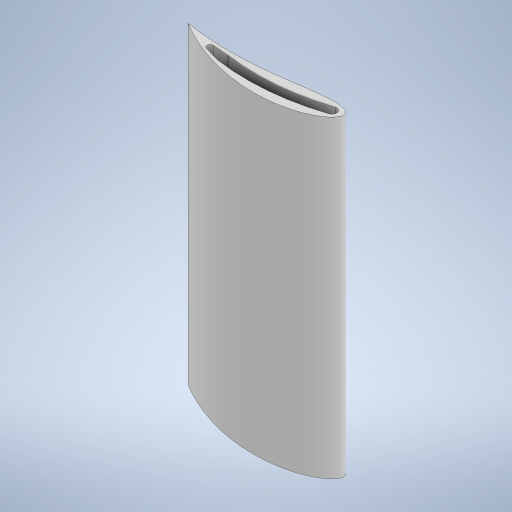
# Autodesk Inventor part: 9518
Saved by Autodesk Inventor 2023 (Build 270158000, 158)
## iProperties
Created: 2023-03-15
Part Number: 9518
Material: 一般
Document SubType Name: Modeling
Designer: USER
Density: 1 g/cm^3
Appearance: 預設
Author: USER
Autodesk Inventor part; units mm, degrees
ref_plane "YZ Plane" through (0, 0, 0) normal (1, 0, 0) x (0, 1, 0)
ref_plane "XZ Plane" through (0, 0, 0) normal (0, 1, 0) x (-1, 0, 0)
ref_plane "XY Plane" through (0, 0, 0) normal (0, 0, 1) x (1, 0, 0)
sketch "草圖1" plane through (0, 0, 0) normal (0, 1, 0) x (-1, 0, 0)
  spline S0 degree 5 poles (50, 0) (50.0018, 0.0049) (49.9549, 0.0322) (49.7247, 0.1379) (49.7279, 0.2103) (49.0894, 0.5065) (48.8341, 0.7267) (48.0356, 1.1334) (47.3779, 1.5287) (46.409, 2.0302) (45.4109, 2.5501) (44.2282, 3.1221) (42.9528, 3.7109) (41.5444, 4.3173) (40.0326, 4.9232) (38.4133, 5.5196) (36.7002, 6.0934) (34.9, 6.6339) (33.0241, 7.1302) (31.0833, 7.572) (29.0901, 7.9505) (27.0573, 8.2573) (24.9994, 8.4858) (22.9309, 8.6309) (20.8674, 8.6883) (18.8247, 8.6569) (16.819, 8.5358) (14.8662, 8.3275) (12.9821, 8.0353) (11.1817, 7.665) (9.4795, 7.2237) (7.8884, 6.7205) (6.42, 6.1652) (5.0847, 5.5689) (3.8908, 4.9431) (2.8449, 4.2994) (1.9517, 3.6485) (1.2135, 3.0004) (0.6319, 2.3616) (0.2072, 1.7375) (-0.0547, 1.1287) (-0.1445, 0.5417) (-0.0431, -0.0146) (0.2327, -0.5065) (0.6667, -0.9034) (1.2361, -1.2172) (1.9287, -1.454) (2.7384, -1.6234) (3.6613, -1.7301) (4.6932, -1.778) (5.8282, -1.7712) (7.0599, -1.7133) (8.3813, -1.6096) (9.7854, -1.4651) (11.2651, -1.2861) (12.8135, -1.0791) (14.4239, -0.8511) (16.0897, -0.6096) (17.8041, -0.3622) (19.5603, -0.1162) (21.3511, 0.121) (23.1691, 0.3426) (25.0059, 0.5429) (26.8531, 0.7166) (28.7012, 0.8597) (30.5403, 0.9698) (32.3598, 1.0451) (34.1488, 1.0857) (35.896, 1.0928) (37.5891, 1.069) (39.2181, 1.0169) (40.7669, 0.9428) (42.2336, 0.8471) (43.5868, 0.7445) (44.856, 0.6222) (45.953, 0.5206) (47.0127, 0.3808) (47.7712, 0.3214) (48.64, 0.1592) (48.9786, 0.1804) (49.6561, 0.0095) (49.7006, 0.0688) (49.9448, 0.0039) (49.9982, -0.0049) (50, 0) knots 0 0 0 0 0 0 0.005631 0.010546 0.017382 0.02568 0.035134 0.045569 0.056859 0.068903 0.081616 0.094923 0.108756 0.123052 0.137755 0.152809 0.168162 0.183765 0.199568 0.215524 0.231585 0.247705 0.263835 0.279929 0.295939 0.311816 0.32751 0.342973 0.358152 0.372996 0.387454 0.401471 0.414995 0.427972 0.440349 0.452078 0.46312 0.473455 0.483105 0.49216 0.500768 0.509124 0.517469 0.526039 0.535015 0.54453 0.554657 0.565407 0.576758 0.588667 0.601088 0.613972 0.627272 0.640942 0.654941 0.669226 0.68376 0.698506 0.713426 0.728485 0.743649 0.75888 0.774142 0.789396 0.804604 0.819723 0.834709 0.849515 0.864091 0.878383 0.892334 0.905881 0.918959 0.931493 0.943401 0.954593 0.96496 0.97437 0.982641 0.989463 0.994372 1 1 1 1 1 1
  point P0 (0, 0)
  point P1 (49.7146, 0.1731)
  point P2 (49.3586, 0.3861)
  point P3 (48.8615, 0.6782)
  point P4 (48.2248, 1.0432)
  point P5 (47.4504, 1.4739)
  point P6 (46.541, 1.9614)
  point P7 (45.4995, 2.496)
  point P8 (44.3301, 3.0669)
  point P9 (43.0373, 3.6629)
  point P10 (41.6267, 4.2721)
  point P11 (40.1046, 4.8827)
  point P12 (38.4784, 5.4828)
  point P13 (36.7563, 6.0603)
  point P14 (34.9477, 6.604)
  point P15 (33.0628, 7.103)
  point P16 (31.1129, 7.5473)
  point P17 (29.1101, 7.9275)
  point P18 (27.0678, 8.2355)
  point P19 (25, 8.4646)
  point P20 (22.9217, 8.6095)
  point P21 (20.8483, 8.6662)
  point P22 (18.7959, 8.633)
  point P23 (16.7807, 8.5097)
  point P24 (14.8189, 8.298)
  point P25 (12.9263, 8.0018)
  point P26 (11.1183, 7.6267)
  point P27 (9.4093, 7.1799)
  point P28 (7.8126, 6.6704)
  point P29 (6.3402, 6.1082)
  point P30 (5.0027, 5.5044)
  point P31 (3.8089, 4.8706)
  point P32 (2.7662, 4.2188)
  point P33 (1.8803, 3.5604)
  point P34 (1.1555, 2.9064)
  point P35 (0.5946, 2.267)
  point P36 (0.1988, 1.6507)
  point P37 (-0.0315, 1.0644)
  point P38 (-0.0972, 0.5131)
  point P39 (0, 0)
  point P40 (0.2513, -0.4578)
  point P41 (0.6471, -0.8441)
  point P42 (1.1827, -1.1602)
  point P43 (1.8527, -1.4076)
  point P44 (2.6505, -1.5884)
  point P45 (3.5694, -1.7054)
  point P46 (4.6018, -1.7617)
  point P47 (5.7403, -1.7612)
  point P48 (6.9771, -1.7083)
  point P49 (8.3044, -1.6082)
  point P50 (9.715, -1.4664)
  point P51 (11.2014, -1.2893)
  point P52 (12.7568, -1.0837)
  point P53 (14.3742, -0.8568)
  point P54 (16.0469, -0.616)
  point P55 (17.7685, -0.3691)
  point P56 (19.5318, -0.1235)
  point P57 (21.33, 0.1136)
  point P58 (23.1554, 0.3352)
  point P59 (25, 0.5354)
  point P60 (26.8552, 0.7091)
  point P61 (28.7116, 0.8523)
  point P62 (30.5594, 0.9623)
  point P63 (32.388, 1.0375)
  point P64 (34.1865, 1.0779)
  point P65 (35.9432, 1.0848)
  point P66 (37.6465, 1.0602)
  point P67 (39.2846, 1.0078)
  point P68 (40.8457, 0.9319)
  point P69 (42.318, 0.8371)
  point P70 (43.6902, 0.7292)
  point P71 (44.9513, 0.6135)
  point P72 (46.0911, 0.4956)
  point P73 (47.0999, 0.3811)
  point P74 (47.9692, 0.2748)
  point P75 (48.6913, 0.1812)
  point P76 (49.26, 0.1043)
  point P77 (49.6698, 0.0472)
  point P78 (49.9173, 0.0119)
  constraints: 80 other
extrude "擠出1" add sketch "草圖1" along normal blind 100
sketch "草圖2" plane through (0, 100, 0) normal (0, 1, 0) x (1, 0, 0)
  arc A0 (-50, 0) -> (0, 0) centre (-25, 64.9885) ccw construction
  arc A1 (-35.0228, -3.9176) -> (-3.0228, -1.0835) centre (-25, 64.9885) ccw construction
  arc A2 (-35.2387, -5.402) -> (-2.5494, -2.5068) centre (-25, 64.9885) ccw
  arc A3 (-34.8069, -2.4332) -> (-3.4962, 0.3398) centre (-25, 64.9885) ccw
  arc A4 (-34.8069, -2.4332) -> (-35.2387, -5.402) centre (-35.0228, -3.9176) ccw
  arc A5 (-2.5494, -2.5068) -> (-3.4962, 0.3398) centre (-3.0228, -1.0835) ccw
  arc A6 (-39.9405, -2.0062) -> (-40.2986, -3.964) centre (-40.0228, -3.0028) ccw
  line L0 (-34.8993, -2.4227) -> (-39.9405, -2.0062)
  line L1 (-35.4366, -5.3594) -> (-40.2986, -3.964)
  dimension "d2" = 1.5
  dimension "d3" = 71.1312
  dimension "d4" = 32
  dimension "d5" = 3.2111
  dimension "d6" = 2
  dimension "d7" = 5
  constraints: 19 point on circle, 8 tangent, 7 centre point, 4 end point, 1 concentric
  measures "d2" radius of A5
  measures "d3" radius of A2
  measures "d4" horizontal distance of A1.start A1.end
  measures "d5" distance of A0.end A1.end
  measures "d6" diameter of A6
  measures "d7" horizontal distance of A1.start A6.centre
extrude "擠出2" cut sketch "草圖2" against normal through all
